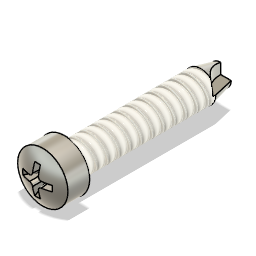
fa6208e3-7742-4840-b170-a1b98c8805f3 (Autodesk Fusion 360 design; units mm, degrees)
description: Tipo I - Parafuso Philips autorroscante de cabeça cilíndrica ASME B18.6.4 3-28 x 0.5 Tipo BT
part number: CRFHTSTBTTI ASME B18.6.4 - 3-28 x 1/2 Aço grau 2 Liso
Autodesk Fusion 360 part; units mm, degrees
sketch "Sketch1" plane through (0, 0, 0) normal (0, 1, 0) x (1, 0, 0)
  line L0 (-1.2573, 0) -> (-1.2573, 12.7)
  line L1 (-1.2573, 12.7) -> (0, 12.7)
  line L2 (0, 12.7) -> (0, -2.413)
  line L3 (-1.2573, 0) -> (-2.0447, 0)
  line L4 (-2.0447, 0) -> (-2.0447, -1.778)
  arc A0 (-2.0447, -1.778) -> (0, -2.413) centre (0, 1.1965) ccw
  dimension "d9" = 2.5146
  dimension "d66" = 4.0894
  dimension "d127" = 2.413
  dimension "d128" = 1.778
  dimension "d129" = 12.7
  constraint perpendicular L0 L1
  constraint perpendicular L0 L3
  constraint coincident origin L3
  constraint vertical L0
  constraint vertical L2
  constraint parallel L2 L4
  constraint coincident L2 A0.centre
  constraint coincident origin L2
  measures "d127" distance of L2.end L3
  measures "d128" distance of L3 L4.end
  measures "d129" distance of origin L1
revolve "Revolve1" add sketch "Sketch1" angle 360 about axis through (0, 0, -12.7) along (0, 0, 1) makes body 1
ref_plane "WorkPlane1" through (0, 0, 2.413) normal (0, 0, 1) x (1, 0, 0)
sketch "Sketch2" plane through (0, 0, 2.413) normal (0, 0, 1) x (1, 0, 0)
  line L0 (-0.2413, -0.2413) -> (-1.3462, -0.2413)
  line L1 (-1.3462, 0.2413) -> (-0.2413, 0.2413)
  line L2 (-1.3462, -0.2413) -> (-1.3462, 0.2413)
  line L3 (-0.2413, -1.3462) -> (-0.2413, -0.2413)
  line L4 (0.2413, -1.3462) -> (-0.2413, -1.3462)
  line L5 (0.2413, -0.2413) -> (0.2413, -1.3462)
  line L6 (1.3462, -0.2413) -> (0.2413, -0.2413)
  line L7 (1.3462, 0.2413) -> (1.3462, -0.2413)
  line L8 (0.2413, 0.2413) -> (1.3462, 0.2413)
  line L9 (0.2413, 1.3462) -> (0.2413, 0.2413)
  line L10 (-0.2413, 1.3462) -> (0.2413, 1.3462)
  line L11 (-0.2413, 0.2413) -> (-0.2413, 1.3462)
  dimension "d137" = 0.4826
  dimension "d139" = 360
  dimension "d140" = 2.6924
  constraint vertical L0.start L1.end
  constraint horizontal L1
  constraint horizontal L0
  constraint coincident L1 L11.start
  constraint coincident L1.end L11.start
  constraint perpendicular L7 L8
  measures "d137" distance of L0.end L1
  measures "d140" distance of L4.start L10
extrude "Extrude3" add sketch "Sketch2" against normal blind 1.397 draft -4 separate body makes body 2
draft "Draft2" angle -30 neutral plane through (0, 0, 2.413) pull (0, 0, 1) 4 faces at (-1.3136, -0.0479, 1.9473) (0.0479, -1.3136, 1.9473) (1.3136, 0.0479, 1.9473) (-0.0479, 1.3136, 1.9473) on bodies 2
fillet "Fillet5" radius 0.2413 4 edges at (-0.1925, -0.1925, 1.7145) (-0.1925, 0.1925, 1.7145) (0.1925, 0.1925, 1.7145) (0.1925, -0.1925, 1.7145) on bodies 2
combine "Combine1" operation cut target body 1 tool bodies 2
thread "Thread1" "Inch Tapping Threads 0.099 3-28 3-28 2B" major diameter 2.4892 minor diameter 1.8542 pitch 0.9071 angle 60 resizes the face on face at (-1.2557, 0.0627, -8.4667) on bodies 1
sketch "Sketch5" plane through (0, 0, 0) normal (0, 1, 0) x (1, 0, 0)
  line L0 (-1.2824, 10.8966) -> (-0.8636, 12.7)
  line L1 (-1.2824, 10.8966) -> (-1.2824, 12.7)
  line L2 (0, 12.7) -> (0, -2.413)
  line L3 (-1.2824, 12.7) -> (0, 12.7)
  dimension "d134" = 1.2824
  dimension "d135" = 1.8034
  dimension "d136" = 0.4188
  constraint coincident L2.start L3.end
  constraint perpendicular L2 L3
  constraint coincident L0.end L3
  constraint perpendicular L1 L3
  measures "d134" distance of L1 L2.start
  measures "d135" distance of L0.start L3
  measures "d136" distance of L0.end L1
revolve "Revolve2" cut sketch "Sketch5" angle 360 about axis through (0, 0, -12.7) along (0, 0, 1) bodies 1
sketch "Sketch8" plane through (0, 0, 0) normal (0, 1, 0) x (1, 0, 0)
  line L0 (0, 12.7) -> (1.2573, 12.7)
  line L1 (1.2573, 12.7) -> (1.2573, 10.8064)
  arc A0 (0, 12.7) -> (1.2573, 10.8064) centre (2.0546, 12.7) ccw
  point P0 (0, 12.7)
  dimension "d132" = 1.2573
  dimension "d133" = 1.8936
  constraint horizontal L0
  constraint perpendicular L0 L1
  constraint coincident P0 L0.start
  constraint coincident L1.end A0.end
  constraint coincident L0 A0.centre
  measures "d132" distance of L1 P0
  measures "d133" distance of L0 L1.end
extrude "Extrude2" cut sketch "Sketch8" along normal blind 1.2573 bodies 1
equation "d9 = adsk_nomdia"
equation "d66 = adsk_headdia"
equation "d71 = adsk_headh"
equation "adsk_nomlen = 0.50 in"
equation "adsk_headh = 0.095 in"
equation "adsk_headdia = 0.161 in"
equation "adsk_nomdia = 0.099 in"
equation "adsk_phildia = 0.106 in"
equation "adsk_philwidth = 0.019 in"
equation "adsk_phildepth = 0.055 in"
equation "adsk_startlen = 0.071 in"
equation "adsk_endpointdia = 0.068 in"
equation "d111 = adsk_nomdia / 2"
equation "d117 = -adsk_phildepth"
equation "adsk_ovalh = 0.025 in"
equation "d127 = adsk_headh"
equation "d128 = adsk_headh - adsk_ovalh"
equation "d129 = adsk_nomlen"
equation "d132 = adsk_nomdia / 2"
equation "d133 = adsk_startlen * 1.05"
equation "d134 = 0.51 * adsk_nomdia"
equation "d135 = adsk_startlen"
equation "d136 = ( adsk_nomdia * 0.51 ) - ( adsk_endpointdia / 2 )"
equation "d137 = adsk_philwidth"
equation "d140 = adsk_phildia"
equation "d142 = adsk_philwidth / 2"
